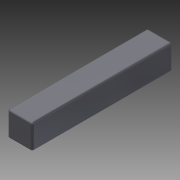
# Autodesk Inventor part: wheel_key
Saved by Autodesk Inventor 2012 (Build 160160000, 160)
## iProperties
Created: 2012-10-25
Part Number: wheel_key
Material: Steel, High Strength Low Alloy
Document SubType Name: Modeling
Designer: Andrew G. Meyer
Mass: 1.39489 g
Surface Area: 2.35372 cm^2
Volume: 0.177919 cm^3
Density: 7.84 g/cm^3
Author: Andrew G. Meyer
Autodesk Inventor part; units mm, degrees
ref_plane "YZ Plane" through (0, 0, 0) normal (1, 0, 0) x (0, 1, 0)
ref_plane "XZ Plane" through (0, 0, 0) normal (0, 1, 0) x (-1, 0, 0)
ref_plane "XY Plane" through (0, 0, 0) normal (0, 0, 1) x (1, 0, 0)
sketch "Sketch1" plane through (0, 0, 0) normal (0, 0, 1) x (1, 0, 0)
  line L0 (-1.5875, 1.5875) -> (1.5875, 1.5875)
  line L1 (1.5875, 1.5875) -> (1.5875, -1.5875)
  line L2 (1.5875, -1.5875) -> (-1.5875, -1.5875)
  line L3 (-1.5875, -1.5875) -> (-1.5875, 1.5875)
  point P0 (0, 0)
  dimension "d0" = 3.175
  dimension "d1" = 3.175
  dimension "d2" = 1.5875
  dimension "d3" = 1.5875
  constraints: 8 end point, 2 parallel, 1 horizontal, 1 perpendicular
  measures "d0" distance of L0.start L0.end
  measures "d1" distance of L2.end L0.start
  measures "d2" distance from line of L0 point (0, 0)
  measures "d3" distance from line of L3 point (0, 0)
extrude "Extrusion1" add sketch "Sketch1" along normal blind 17.78
fillet "Fillet1" radius 0.254 12 edges at (1.5875, 1.5875, 8.89) (-1.5875, 1.5875, 8.89) (-1.5875, -1.5875, 8.89) (1.5875, -1.5875, 8.89) (0, -1.5875, 17.78) (1.5875, 0, 17.78) (0, 1.5875, 17.78) (-1.5875, 0, 17.78) (0, 1.5875, 0) (-1.5875, 0, 0) (0, -1.5875, 0) (1.5875, 0, 0)
equation "\"d1\" = d0"
equation "\"d2\" = 0.5 * d1"
equation "\"d3\" = 0.5 * d0"
body "Solid1"
